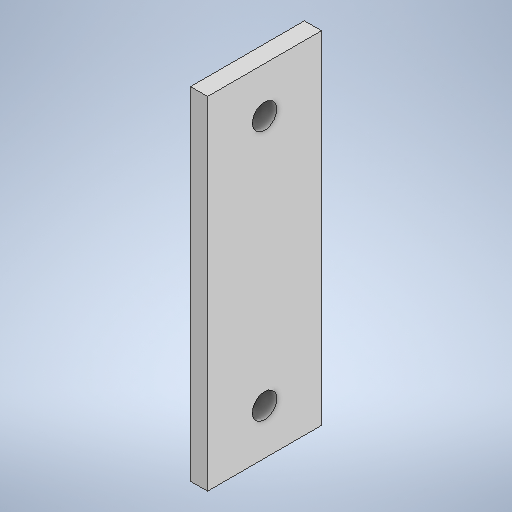
# Autodesk Inventor part: BedBeltMount2
Saved by Autodesk Inventor 2025.2 (Build 292293000, 293)
## iProperties
Created: 2025-07-28
Part Number: BedBeltMount2
Material: Generic
Document SubType Name: Modeling
Designer: Simon
Density: 1 g/cm^3
Appearance: Default
Author: Simon
Autodesk Inventor part; units mm, degrees
ref_plane "YZ Plane" through (0, 0, 0) normal (1, 0, 0) x (0, 1, 0)
ref_plane "XZ Plane" through (0, 0, 0) normal (0, 1, 0) x (-1, 0, 0)
ref_plane "XY Plane" through (0, 0, 0) normal (0, 0, 1) x (1, 0, 0)
sketch "Sketch1" plane through (0, 0, 0) normal (1, 0, 0) x (0, 1, 0)
  line L0 (0, 0) -> (60, 0)
  line L1 (60, 0) -> (60, 20)
  line L2 (60, 20) -> (0, 20)
  line L3 (0, 20) -> (0, 0)
  line L4 (0, 10) -> (8, 10)
  line L5 (60, 10) -> (52, 10)
  circle A0 centre (52, 10) radius 2.15
  circle A1 centre (8, 10) radius 2.15
  dimension "d0" = 60
  dimension "d1" = 20
  dimension "d2" = 8
  dimension "d3" = 8
  dimension "d4" = 4.3
  dimension "d5" = 4.3
  constraints: 12 end point, 2 centre point, 2 coincident, 2 horizontal, 2 midpoint, 2 parallel, 2 perpendicular
  measures "d0" distance of L2.end L1.end
  measures "d1" distance of L1.end L0.end
  measures "d2" distance of L4.start L4.end
  measures "d3" distance of L5.start L5.end
  measures "d4" diameter of A0
  measures "d5" diameter of A1
extrude "Extrusion1" add sketch "Sketch1" along normal blind 3
body "Solid1"
